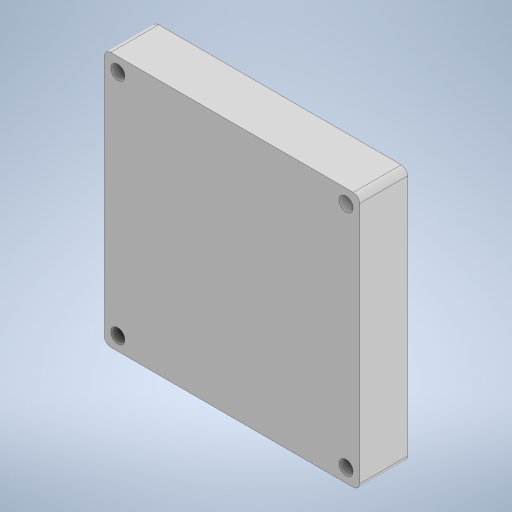
# Autodesk Inventor part: FAN SPACE MODEL
Saved by Autodesk Inventor 2023 (Build 270158000, 158)
## iProperties
Created: 2023-03-17
Part Number: FAN SPACE MODEL
Material: Generic
Document SubType Name: Modeling
Designer: Louis
Density: 1 g/cm^3
Appearance: Default
Author: Louis
Autodesk Inventor part; units mm, degrees
ref_plane "YZ Plane" through (0, 0, 0) normal (1, 0, 0) x (0, 1, 0)
ref_plane "XZ Plane" through (0, 0, 0) normal (0, 1, 0) x (-1, 0, 0)
ref_plane "XY Plane" through (0, 0, 0) normal (0, 0, 1) x (1, 0, 0)
sketch "Sketch1" plane through (0, 0, 0) normal (0, 0, 1) x (1, 0, 0)
  line L0 (-40, 40) -> (40, 40)
  line L1 (40, 40) -> (40, -40)
  line L2 (40, -40) -> (-40, -40)
  line L3 (-40, -40) -> (-40, 40)
  point P0 (0, 0)
  point P1 (0, 40)
  point P2 (-40, 0)
  dimension "d0" = 80
  constraints: 8 end point, 2 midpoint, 2 parallel, 2 perpendicular, 1 horizontal, 1 horizontal alignment, 1 vertical alignment
  measures "d0" distance of L0.start L0.end
extrude "Extrusion1" add sketch "Sketch1" along normal blind 15
sketch "Sketch2" plane through (0, 0, 15) normal (0, 0, 1) x (1, 0, 0)
  line L0 (-35.75, 35.75) -> (35.75, 35.75)
  line L1 (35.75, 35.75) -> (35.75, -35.75)
  line L2 (35.75, -35.75) -> (-35.75, -35.75)
  line L3 (-35.75, -35.75) -> (-35.75, 35.75)
  point P0 (0, 0)
  point P1 (0, 35.75)
  point P2 (-35.75, 0)
  dimension "d3" = 71.5
  constraints: 8 end point, 4 coincident, 2 midpoint, 2 parallel, 2 perpendicular, 1 horizontal, 1 horizontal alignment, 1 vertical alignment
  measures "d3" distance of L0.start L0.end
hole "Hole1" at (-35.75, 35.75, 15) at (35.75, 35.75, 15) at (-35.75, -35.75, 15) at (35.75, -35.75, 15) direction (0, 0, -1) diameter 4.4 end through all
fillet "Fillet1" radius 2 4 edges at (-40, 40, 7.5) (40, 40, 7.5) (40, -40, 7.5) (-40, -40, 7.5)
body "Solid1"
